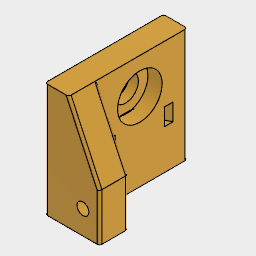
Y_End_Stop_Bracket_F01 (Autodesk Fusion 360 design; units mm, degrees)
Autodesk Fusion 360 part; units mm, degrees
note: some values were not read from the file. Set by a fixed rule: which sketch regions a step uses.
sketch "スケッチ1" plane through (0, 0, 0) normal (0, 0, 1) x (1, 0, 0)
  line L0 (0, 10) -> (-5, 10)
  line L1 (-5, 10) -> (-5, -15)
  line L2 (-5, -15) -> (0, -15)
  line L3 (0, -15) -> (0, 10)
  dimension "d1" = 25
  dimension "d2" = 5
  dimension "d3" = 10
  measures "d1" distance of L0.start L2.end
  measures "d2" distance of L0.start L0.end
  measures "d3" distance of origin L0
extrude "押し出し1" add sketch "スケッチ1" against normal blind 24
sketch "スケッチ2" plane through (0, 0, 0) normal (1, 0, 0) x (0, 1, 0)
  line L0 (10, 0) -> (-15, 0)
  line L1 (-15, 0) -> (-15, -24)
  line L2 (-15, -24) -> (10, -24)
  line L3 (10, -24) -> (10, 0)
  line L4 (0, 0) -> (0, -24) construction
  circle A0 centre (0, -7.5) radius 2.7
  circle A1 centre (0, -7.5) radius 4.7
  line L5 (-9, 0) -> (-9, -24)
  line L6 (-15, -14) -> (-9, -14)
  line L7 (-4, -24) -> (-4, -12.5)
  line L8 (-4, -12.5) -> (4, -12.5)
  line L9 (4, -12.5) -> (4, -24)
  dimension "d6" = 5.4
  dimension "d7" = 9.4
  dimension "d8" = 7.5
  dimension "d9" = 6
  dimension "d10" = 10
  dimension "d19" = 8
  dimension "d20" = 4
  dimension "d21" = 11.5
  measures "d6" diameter of A0
  measures "d7" diameter of A1
  measures "d8" distance of L0 A0.centre
  measures "d9" distance of L1 L5
  measures "d10" distance of L2 L6
  measures "d19" distance of L7 L9
  measures "d20" distance of L4.end L7
  measures "d21" distance of L8.end L9.end
extrude "押し出し2" cut sketch "スケッチ2" against normal up to surface (5 mm away) contours A0
extrude "押し出し3" cut sketch "スケッチ2" against normal blind 3 contours A1
extrude "押し出し4" add sketch "スケッチ2" along normal blind 6.5 contours L1 L2 L5 L6
chamfer "面取り1" distance 14 distance2 6.5 1 edges at (0, -12, -14) measured on face at (0, 0.4504, -20.0623)
extrude "押し出し5" add sketch "スケッチ2" against normal blind 6.5 contours L2 L7 L8 L9
sketch "スケッチ3" plane through (0, 0, 0) normal (0, 0, 1) x (-1, 0, 0)
  line L0 (0, 15) -> (0, 9)
  line L1 (0, 9) -> (0, -10)
  line L2 (0, -10) -> (5, -10)
  line L3 (5, -10) -> (5, 15)
  line L4 (5, 15) -> (0, 15)
  line L5 (0, 0) -> (-3, 0) construction
  circle A0 centre (-3, 0) radius 7.6
  circle A1 centre (-3, 0) radius 6
  dimension "d24" = 3
  dimension "d25" = 15.2
  dimension "d26" = 12
  measures "d24" distance of L5.start L5.end
  measures "d25" diameter of A0
  measures "d26" diameter of A1
extrude "押し出し6" cut sketch "スケッチ3" against normal blind 3.6 from surface at -12 contours L1 A0 A1 picked at (0.3272, 6.2175)
hole "穴1" at (3, -15, -19) direction (0, 1, 0) diameter 2.5 depth 6 tip angle 118
fillet "フィレット1" radius 0.5 7 edges at (-5, 10, -12) (0, 10, -12) (3.25, -9, -7) (6.5, -9, -19) (3.25, -15, -7) (6.5, -15, -19) (-5, -15, -12)
equation "d20 = d19 / 2"
